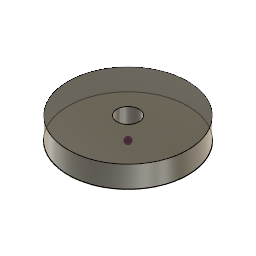
2-Roller_Insert v1 (Autodesk Fusion 360 design; units mm, degrees)
Autodesk Fusion 360 part; units mm, degrees
sketch "Roller_Insert" plane through (0, 0, 0) normal (0, 0, 1) x (1, 0, 0)
  circle A0 centre (0, 0) radius 349.25
  dimension "d1" = 698.5
  measures "d1" diameter of A0
extrude "Extrude1" add sketch "Roller_Insert" along normal blind 127
hole "Hole1" at (0, 0, 127) direction (0, 0, -1) diameter 129 end through all
